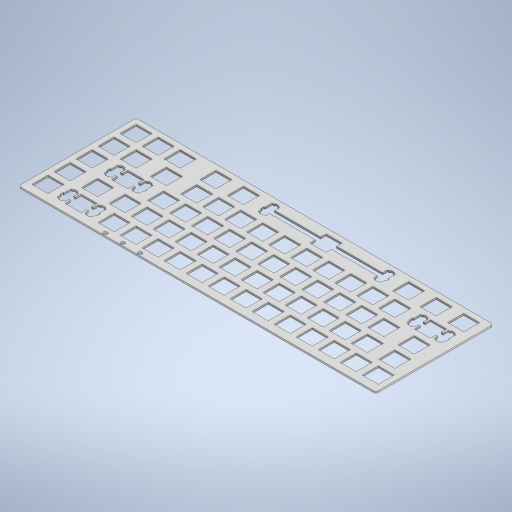
# Autodesk Inventor part: case_plate_p1
Saved by Autodesk Inventor 2024 (Build 280153000, 153)
## iProperties
Created: 2023-08-02
Part Number: case_plate_p1
Material: Generic
Document SubType Name: Modeling
Designer: Mika
Density: 1 g/cm^3
Appearance: Default
Author: Mika
Autodesk Inventor part; units mm, degrees
ref_plane "YZ Plane" through (0, 0, 0) normal (1, 0, 0) x (0, 1, 0)
ref_plane "XZ Plane" through (0, 0, 0) normal (0, 1, 0) x (-1, 0, 0)
ref_plane "XY Plane" through (0, 0, 0) normal (0, 0, 1) x (1, 0, 0)
sketch "Sketch1" plane through (0, 0, 0) normal (0, 1, 0) x (-1, 0, 0)
  line L0 (309.0479, 99.8402) -> (309.0479, 2.3404)
  line L1 (307.045, 0.3402) -> (2.0931, 0.3389)
  line L2 (0.096, 2.3404) -> (0.096, 99.8389)
  line L3 (2.096, 101.8389) -> (307.045, 101.8402)
  line L4 (126.213, 18.8654) -> (126.213, 14.1663)
  line L5 (126.213, 14.1663) -> (86.4387, 14.1663)
  line L6 (86.4387, 14.1663) -> (86.4387, 17.395)
  line L7 (86.4387, 17.395) -> (84.7136, 17.395)
  line L8 (84.7136, 17.395) -> (84.7136, 18.3155)
  line L9 (84.7136, 18.3155) -> (81.5633, 18.3155)
  line L10 (81.5633, 18.3155) -> (81.5633, 17.395)
  line L11 (81.5633, 17.395) -> (79.8382, 17.395)
  line L12 (79.8382, 17.395) -> (79.8382, 14.1663)
  line L13 (79.8382, 14.1663) -> (79.0141, 14.1663)
  line L14 (79.0141, 14.1663) -> (79.0141, 11.5163)
  line L15 (79.0141, 11.5163) -> (79.8382, 11.5163)
  line L16 (79.8382, 11.5163) -> (79.8382, 5.2462)
  line L17 (79.8382, 5.2462) -> (81.5633, 5.2462)
  line L18 (81.5633, 5.2462) -> (81.5633, 4.265)
  line L19 (81.5633, 4.265) -> (84.7136, 4.265)
  line L20 (84.7136, 4.265) -> (84.7136, 5.2462)
  line L21 (84.7136, 5.2462) -> (86.4387, 5.2462)
  line L22 (86.4387, 5.2462) -> (86.4387, 9.7166)
  line L23 (86.4387, 9.7166) -> (126.213, 9.7166)
  line L24 (126.213, 9.7166) -> (126.213, 5.0161)
  line L25 (126.213, 5.0161) -> (140.064, 5.0161)
  line L26 (140.064, 5.0161) -> (140.064, 9.7166)
  line L27 (140.064, 9.7166) -> (179.838, 9.7166)
  line L28 (179.838, 9.7166) -> (179.838, 5.2462)
  line L29 (179.838, 5.2462) -> (181.563, 5.2462)
  line L30 (181.563, 5.2462) -> (181.563, 4.265)
  line L31 (181.563, 4.265) -> (184.714, 4.265)
  line L32 (184.714, 4.265) -> (184.714, 5.2462)
  line L33 (184.714, 5.2462) -> (186.439, 5.2462)
  line L34 (186.439, 5.2462) -> (186.439, 11.5163)
  line L35 (186.439, 11.5163) -> (187.263, 11.5163)
  line L36 (187.263, 11.5163) -> (187.263, 14.1663)
  line L37 (187.263, 14.1663) -> (186.439, 14.1663)
  line L38 (186.439, 14.1663) -> (186.439, 17.395)
  line L39 (186.439, 17.395) -> (184.714, 17.395)
  line L40 (184.714, 17.395) -> (184.714, 18.3155)
  line L41 (184.714, 18.3155) -> (181.563, 18.3155)
  line L42 (181.563, 18.3155) -> (181.563, 17.395)
  line L43 (181.563, 17.395) -> (179.838, 17.395)
  line L44 (179.838, 17.395) -> (179.838, 14.1663)
  line L45 (179.838, 14.1663) -> (140.064, 14.1663)
  line L46 (140.064, 14.1663) -> (140.064, 18.8654)
  line L47 (140.064, 18.8654) -> (126.213, 18.8654)
  line L48 (7.152, 18.8654) -> (21.0013, 18.8654)
  line L49 (21.0013, 18.8654) -> (21.0013, 5.0161)
  line L50 (21.0013, 5.0161) -> (7.152, 5.0161)
  line L51 (7.152, 5.0161) -> (7.152, 18.8654)
  line L52 (30.9631, 18.8654) -> (44.8137, 18.8654)
  line L53 (44.8137, 18.8654) -> (44.8137, 5.0161)
  line L54 (44.8137, 5.0161) -> (30.9631, 5.0161)
  line L55 (30.9631, 5.0161) -> (30.9631, 18.8654)
  line L56 (54.7769, 18.8654) -> (68.6262, 18.8654)
  line L57 (68.6262, 18.8654) -> (68.6262, 5.0161)
  line L58 (68.6262, 5.0161) -> (54.7769, 5.0161)
  line L59 (54.7769, 5.0161) -> (54.7769, 18.8654)
  line L60 (197.652, 18.8654) -> (211.501, 18.8654)
  line L61 (211.501, 18.8654) -> (211.501, 5.0161)
  line L62 (211.501, 5.0161) -> (197.652, 5.0161)
  line L63 (197.652, 5.0161) -> (197.652, 18.8654)
  line L64 (221.463, 18.8654) -> (235.314, 18.8654)
  line L65 (235.314, 18.8654) -> (235.314, 5.0161)
  line L66 (235.314, 5.0161) -> (221.463, 5.0161)
  line L67 (221.463, 5.0161) -> (221.463, 18.8654)
  line L68 (252.421, 18.8654) -> (266.27, 18.8654)
  line L69 (266.27, 18.8654) -> (266.27, 5.0161)
  line L70 (266.27, 5.0161) -> (252.421, 5.0161)
  line L71 (252.421, 5.0161) -> (252.421, 18.8654)
  line L72 (271.471, 18.8654) -> (285.32, 18.8654)
  line L73 (285.32, 18.8654) -> (285.32, 5.0161)
  line L74 (285.32, 5.0161) -> (271.471, 5.0161)
  line L75 (271.471, 5.0161) -> (271.471, 18.8654)
  line L76 (290.521, 18.8654) -> (304.37, 18.8654)
  line L77 (304.37, 18.8654) -> (304.37, 5.0161)
  line L78 (304.37, 5.0161) -> (290.521, 5.0161)
  line L79 (290.521, 5.0161) -> (290.521, 18.8654)
  line L80 (16.677, 37.9155) -> (16.677, 33.2163)
  line L81 (16.677, 33.2163) -> (15.0013, 33.2163)
  line L82 (15.0013, 33.2163) -> (15.0013, 36.4451)
  line L83 (15.0013, 36.4451) -> (13.276, 36.4451)
  line L84 (13.276, 36.4451) -> (13.276, 37.3655)
  line L85 (13.276, 37.3655) -> (10.1258, 37.3655)
  line L86 (10.1258, 37.3655) -> (10.1258, 36.4451)
  line L87 (10.1258, 36.4451) -> (8.4019, 36.4451)
  line L88 (8.4019, 36.4451) -> (8.4019, 33.2163)
  line L89 (8.4019, 33.2163) -> (7.5765, 33.2163)
  line L90 (7.5765, 33.2163) -> (7.5765, 30.5663)
  line L91 (7.5765, 30.5663) -> (8.4019, 30.5663)
  line L92 (8.4019, 30.5663) -> (8.4019, 24.2962)
  line L93 (8.4019, 24.2962) -> (10.1258, 24.2962)
  line L94 (10.1258, 24.2962) -> (10.1258, 23.315)
  line L95 (10.1258, 23.315) -> (13.276, 23.315)
  line L96 (13.276, 23.315) -> (13.276, 24.2962)
  line L97 (13.276, 24.2962) -> (15.0013, 24.2962)
  line L98 (15.0013, 24.2962) -> (15.0013, 28.7652)
  line L99 (15.0013, 28.7652) -> (16.677, 28.7652)
  line L100 (16.677, 28.7652) -> (16.677, 24.0661)
  line L101 (16.677, 24.0661) -> (30.5263, 24.0661)
  line L102 (30.5263, 24.0661) -> (30.5263, 28.7652)
  line L103 (30.5263, 28.7652) -> (32.202, 28.7652)
  line L104 (32.202, 28.7652) -> (32.202, 24.2962)
  line L105 (32.202, 24.2962) -> (33.9259, 24.2962)
  line L106 (33.9259, 24.2962) -> (33.9259, 23.315)
  line L107 (33.9259, 23.315) -> (37.0762, 23.315)
  line L108 (37.0762, 23.315) -> (37.0762, 24.2962)
  line L109 (37.0762, 24.2962) -> (38.8013, 24.2962)
  line L110 (38.8013, 24.2962) -> (38.8013, 30.5663)
  line L111 (38.8013, 30.5663) -> (39.6268, 30.5663)
  line L112 (39.6268, 30.5663) -> (39.6268, 33.2163)
  line L113 (39.6268, 33.2163) -> (38.8013, 33.2163)
  line L114 (38.8013, 33.2163) -> (38.8013, 36.4451)
  line L115 (38.8013, 36.4451) -> (37.0762, 36.4451)
  line L116 (37.0762, 36.4451) -> (37.0762, 37.3655)
  line L117 (37.0762, 37.3655) -> (33.9259, 37.3655)
  line L118 (33.9259, 37.3655) -> (33.9259, 36.4451)
  line L119 (33.9259, 36.4451) -> (32.202, 36.4451)
  line L120 (32.202, 36.4451) -> (32.202, 33.2163)
  line L121 (32.202, 33.2163) -> (30.5263, 33.2163)
  line L122 (30.5263, 33.2163) -> (30.5263, 37.9155)
  line L123 (30.5263, 37.9155) -> (16.677, 37.9155)
  line L124 (47.6321, 37.9155) -> (61.4825, 37.9155)
  line L125 (61.4825, 37.9155) -> (61.4825, 24.0661)
  line L126 (61.4825, 24.0661) -> (47.6321, 24.0661)
  line L127 (47.6321, 24.0661) -> (47.6321, 37.9155)
  line L128 (66.6821, 37.9155) -> (80.5325, 37.9155)
  line L129 (80.5325, 37.9155) -> (80.5325, 24.0661)
  line L130 (80.5325, 24.0661) -> (66.6821, 24.0661)
  line L131 (66.6821, 24.0661) -> (66.6821, 37.9155)
  line L132 (85.7321, 37.9155) -> (99.5825, 37.9155)
  line L133 (99.5825, 37.9155) -> (99.5825, 24.0661)
  line L134 (99.5825, 24.0661) -> (85.7321, 24.0661)
  line L135 (85.7321, 24.0661) -> (85.7321, 37.9155)
  line L136 (104.782, 37.9155) -> (118.632, 37.9155)
  line L137 (118.632, 37.9155) -> (118.632, 24.0661)
  line L138 (118.632, 24.0661) -> (104.782, 24.0661)
  line L139 (104.782, 24.0661) -> (104.782, 37.9155)
  line L140 (123.832, 37.9155) -> (137.682, 37.9155)
  line L141 (137.682, 37.9155) -> (137.682, 24.0661)
  line L142 (137.682, 24.0661) -> (123.832, 24.0661)
  line L143 (123.832, 24.0661) -> (123.832, 37.9155)
  line L144 (142.882, 37.9155) -> (156.732, 37.9155)
  line L145 (156.732, 37.9155) -> (156.732, 24.0661)
  line L146 (156.732, 24.0661) -> (142.882, 24.0661)
  line L147 (142.882, 24.0661) -> (142.882, 37.9155)
  line L148 (161.932, 37.9155) -> (175.782, 37.9155)
  line L149 (175.782, 37.9155) -> (175.782, 24.0661)
  line L150 (175.782, 24.0661) -> (161.932, 24.0661)
  line L151 (161.932, 24.0661) -> (161.932, 37.9155)
  line L152 (180.982, 37.9155) -> (194.832, 37.9155)
  line L153 (194.832, 37.9155) -> (194.832, 24.0661)
  line L154 (194.832, 24.0661) -> (180.982, 24.0661)
  line L155 (180.982, 24.0661) -> (180.982, 37.9155)
  line L156 (200.032, 37.9155) -> (213.882, 37.9155)
  line L157 (213.882, 37.9155) -> (213.882, 24.0661)
  line L158 (213.882, 24.0661) -> (200.032, 24.0661)
  line L159 (200.032, 24.0661) -> (200.032, 37.9155)
  line L160 (219.082, 37.9155) -> (232.932, 37.9155)
  line L161 (232.932, 37.9155) -> (232.932, 24.0661)
  line L162 (232.932, 24.0661) -> (219.082, 24.0661)
  line L163 (219.082, 24.0661) -> (219.082, 37.9155)
  line L164 (245.277, 37.9155) -> (259.126, 37.9155)
  line L165 (259.126, 37.9155) -> (259.126, 24.0661)
  line L166 (259.126, 24.0661) -> (245.277, 24.0661)
  line L167 (245.277, 24.0661) -> (245.277, 37.9155)
  line L168 (271.471, 37.9155) -> (285.32, 37.9155)
  line L169 (285.32, 37.9155) -> (285.32, 24.0661)
  line L170 (285.32, 24.0661) -> (271.471, 24.0661)
  line L171 (271.471, 24.0661) -> (271.471, 37.9155)
  line L172 (290.521, 37.9155) -> (304.37, 37.9155)
  line L173 (304.37, 37.9155) -> (304.37, 24.0661)
  line L174 (304.37, 24.0661) -> (290.521, 24.0661)
  line L175 (290.521, 24.0661) -> (290.521, 37.9155)
  line L176 (259.563, 56.9655) -> (259.563, 52.2661)
  line L177 (259.563, 52.2661) -> (257.889, 52.2661)
  line L178 (257.889, 52.2661) -> (257.889, 55.4951)
  line L179 (257.889, 55.4951) -> (256.162, 55.4951)
  line L180 (256.162, 55.4951) -> (256.162, 56.4155)
  line L181 (256.162, 56.4155) -> (253.013, 56.4155)
  line L182 (253.013, 56.4155) -> (253.013, 55.4951)
  line L183 (253.013, 55.4951) -> (251.288, 55.4951)
  line L184 (251.288, 55.4951) -> (251.288, 52.2661)
  line L185 (251.288, 52.2661) -> (250.464, 52.2661)
  line L186 (250.464, 52.2661) -> (250.464, 49.6164)
  line L187 (250.464, 49.6164) -> (251.288, 49.6164)
  line L188 (251.288, 49.6164) -> (251.288, 43.3462)
  line L189 (251.288, 43.3462) -> (253.013, 43.3462)
  line L190 (253.013, 43.3462) -> (253.013, 42.3651)
  line L191 (253.013, 42.3651) -> (256.162, 42.3651)
  line L192 (256.162, 42.3651) -> (256.162, 43.3462)
  line L193 (256.162, 43.3462) -> (257.889, 43.3462)
  line L194 (257.889, 43.3462) -> (257.889, 47.8151)
  line L195 (257.889, 47.8151) -> (259.563, 47.8151)
  line L196 (259.563, 47.8151) -> (259.563, 43.1161)
  line L197 (259.563, 43.1161) -> (273.414, 43.1161)
  line L198 (273.414, 43.1161) -> (273.414, 47.8151)
  line L199 (273.414, 47.8151) -> (275.088, 47.8151)
  line L200 (275.088, 47.8151) -> (275.088, 43.3462)
  line L201 (275.088, 43.3462) -> (276.813, 43.3462)
  line L202 (276.813, 43.3462) -> (276.813, 42.3651)
  line L203 (276.813, 42.3651) -> (279.964, 42.3651)
  line L204 (279.964, 42.3651) -> (279.964, 43.3462)
  line L205 (279.964, 43.3462) -> (281.689, 43.3462)
  line L206 (281.689, 43.3462) -> (281.689, 49.6164)
  line L207 (281.689, 49.6164) -> (282.513, 49.6164)
  line L208 (282.513, 49.6164) -> (282.513, 52.2661)
  line L209 (282.513, 52.2661) -> (281.689, 52.2661)
  line L210 (281.689, 52.2661) -> (281.689, 55.4951)
  line L211 (281.689, 55.4951) -> (279.964, 55.4951)
  line L212 (279.964, 55.4951) -> (279.964, 56.4155)
  line L213 (279.964, 56.4155) -> (276.813, 56.4155)
  line L214 (276.813, 56.4155) -> (276.813, 55.4951)
  line L215 (276.813, 55.4951) -> (275.088, 55.4951)
  line L216 (275.088, 55.4951) -> (275.088, 52.2661)
  line L217 (275.088, 52.2661) -> (273.414, 52.2661)
  line L218 (273.414, 52.2661) -> (273.414, 56.9655)
  line L219 (273.414, 56.9655) -> (259.563, 56.9655)
  line L220 (11.9131, 56.9655) -> (25.7638, 56.9655)
  line L221 (25.7638, 56.9655) -> (25.7638, 43.1161)
  line L222 (25.7638, 43.1161) -> (11.9131, 43.1161)
  line L223 (11.9131, 43.1161) -> (11.9131, 56.9655)
  line L224 (38.1071, 56.9655) -> (51.9575, 56.9655)
  line L225 (51.9575, 56.9655) -> (51.9575, 43.1161)
  line L226 (51.9575, 43.1161) -> (38.1071, 43.1161)
  line L227 (38.1071, 43.1161) -> (38.1071, 56.9655)
  line L228 (57.1571, 56.9655) -> (71.0075, 56.9655)
  line L229 (71.0075, 56.9655) -> (71.0075, 43.1161)
  line L230 (71.0075, 43.1161) -> (57.1571, 43.1161)
  line L231 (57.1571, 43.1161) -> (57.1571, 56.9655)
  line L232 (76.2071, 56.9655) -> (90.0575, 56.9655)
  line L233 (90.0575, 56.9655) -> (90.0575, 43.1161)
  line L234 (90.0575, 43.1161) -> (76.2071, 43.1161)
  line L235 (76.2071, 43.1161) -> (76.2071, 56.9655)
  line L236 (95.2571, 56.9655) -> (109.107, 56.9655)
  line L237 (109.107, 56.9655) -> (109.107, 43.1161)
  line L238 (109.107, 43.1161) -> (95.2571, 43.1161)
  line L239 (95.2571, 43.1161) -> (95.2571, 56.9655)
  line L240 (114.307, 56.9655) -> (128.157, 56.9655)
  line L241 (128.157, 56.9655) -> (128.157, 43.1161)
  line L242 (128.157, 43.1161) -> (114.307, 43.1161)
  line L243 (114.307, 43.1161) -> (114.307, 56.9655)
  line L244 (133.357, 56.9655) -> (147.207, 56.9655)
  line L245 (147.207, 56.9655) -> (147.207, 43.1161)
  line L246 (147.207, 43.1161) -> (133.357, 43.1161)
  line L247 (133.357, 43.1161) -> (133.357, 56.9655)
  line L248 (152.407, 56.9655) -> (166.257, 56.9655)
  line L249 (166.257, 56.9655) -> (166.257, 43.1161)
  line L250 (166.257, 43.1161) -> (152.407, 43.1161)
  line L251 (152.407, 43.1161) -> (152.407, 56.9655)
  line L252 (171.457, 56.9655) -> (185.307, 56.9655)
  line L253 (185.307, 56.9655) -> (185.307, 43.1161)
  line L254 (185.307, 43.1161) -> (171.457, 43.1161)
  line L255 (171.457, 43.1161) -> (171.457, 56.9655)
  line L256 (190.507, 56.9655) -> (204.357, 56.9655)
  line L257 (204.357, 56.9655) -> (204.357, 43.1161)
  line L258 (204.357, 43.1161) -> (190.507, 43.1161)
  line L259 (190.507, 43.1161) -> (190.507, 56.9655)
  line L260 (209.557, 56.9655) -> (223.407, 56.9655)
  line L261 (223.407, 56.9655) -> (223.407, 43.1161)
  line L262 (223.407, 43.1161) -> (209.557, 43.1161)
  line L263 (209.557, 43.1161) -> (209.557, 56.9655)
  line L264 (228.607, 56.9655) -> (242.457, 56.9655)
  line L265 (242.457, 56.9655) -> (242.457, 43.1161)
  line L266 (242.457, 43.1161) -> (228.607, 43.1161)
  line L267 (228.607, 43.1161) -> (228.607, 56.9655)
  line L268 (290.521, 56.9655) -> (304.37, 56.9655)
  line L269 (304.37, 56.9655) -> (304.37, 43.1161)
  line L270 (304.37, 43.1161) -> (290.521, 43.1161)
  line L271 (290.521, 43.1161) -> (290.521, 56.9655)
  line L272 (9.5319, 76.0155) -> (23.3826, 76.0155)
  line L273 (23.3826, 76.0155) -> (23.3826, 62.1661)
  line L274 (23.3826, 62.1661) -> (9.5319, 62.1661)
  line L275 (9.5319, 62.1661) -> (9.5319, 76.0155)
  line L276 (33.3458, 76.0155) -> (47.195, 76.0155)
  line L277 (47.195, 76.0155) -> (47.195, 62.1661)
  line L278 (47.195, 62.1661) -> (33.3458, 62.1661)
  line L279 (33.3458, 62.1661) -> (33.3458, 76.0155)
  line L280 (52.3956, 76.0155) -> (66.245, 76.0155)
  line L281 (66.245, 76.0155) -> (66.245, 62.1661)
  line L282 (66.245, 62.1661) -> (52.3956, 62.1661)
  line L283 (52.3956, 62.1661) -> (52.3956, 76.0155)
  line L284 (71.4456, 76.0155) -> (85.295, 76.0155)
  line L285 (85.295, 76.0155) -> (85.295, 62.1661)
  line L286 (85.295, 62.1661) -> (71.4456, 62.1661)
  line L287 (71.4456, 62.1661) -> (71.4456, 76.0155)
  line L288 (90.4946, 76.0155) -> (104.345, 76.0155)
  line L289 (104.345, 76.0155) -> (104.345, 62.1661)
  line L290 (104.345, 62.1661) -> (90.4946, 62.1661)
  line L291 (90.4946, 62.1661) -> (90.4946, 76.0155)
  line L292 (109.545, 76.0155) -> (123.395, 76.0155)
  line L293 (123.395, 76.0155) -> (123.395, 62.1661)
  line L294 (123.395, 62.1661) -> (109.545, 62.1661)
  line L295 (109.545, 62.1661) -> (109.545, 76.0155)
  line L296 (128.595, 76.0155) -> (142.445, 76.0155)
  line L297 (142.445, 76.0155) -> (142.445, 62.1661)
  line L298 (142.445, 62.1661) -> (128.595, 62.1661)
  line L299 (128.595, 62.1661) -> (128.595, 76.0155)
  line L300 (147.645, 76.0155) -> (161.495, 76.0155)
  line L301 (161.495, 76.0155) -> (161.495, 62.1661)
  line L302 (161.495, 62.1661) -> (147.645, 62.1661)
  line L303 (147.645, 62.1661) -> (147.645, 76.0155)
  line L304 (166.696, 76.0155) -> (180.545, 76.0155)
  line L305 (180.545, 76.0155) -> (180.545, 62.1661)
  line L306 (180.545, 62.1661) -> (166.696, 62.1661)
  line L307 (166.696, 62.1661) -> (166.696, 76.0155)
  line L308 (185.746, 76.0155) -> (199.595, 76.0155)
  line L309 (199.595, 76.0155) -> (199.595, 62.1661)
  line L310 (199.595, 62.1661) -> (185.746, 62.1661)
  line L311 (185.746, 62.1661) -> (185.746, 76.0155)
  line L312 (204.796, 76.0155) -> (218.645, 76.0155)
  line L313 (218.645, 76.0155) -> (218.645, 62.1661)
  line L314 (218.645, 62.1661) -> (204.796, 62.1661)
  line L315 (204.796, 62.1661) -> (204.796, 76.0155)
  line L316 (223.846, 76.0155) -> (237.695, 76.0155)
  line L317 (237.695, 76.0155) -> (237.695, 62.1661)
  line L318 (237.695, 62.1661) -> (223.846, 62.1661)
  line L319 (223.846, 62.1661) -> (223.846, 76.0155)
  line L320 (242.896, 76.0155) -> (256.745, 76.0155)
  line L321 (256.745, 76.0155) -> (256.745, 62.1661)
  line L322 (256.745, 62.1661) -> (242.896, 62.1661)
  line L323 (242.896, 62.1661) -> (242.896, 76.0155)
  line L324 (266.707, 76.0155) -> (280.557, 76.0155)
  line L325 (280.557, 76.0155) -> (280.557, 62.1661)
  line L326 (280.557, 62.1661) -> (266.707, 62.1661)
  line L327 (266.707, 62.1661) -> (266.707, 76.0155)
  line L328 (290.521, 76.0155) -> (304.37, 76.0155)
  line L329 (304.37, 76.0155) -> (304.37, 62.1661)
  line L330 (304.37, 62.1661) -> (290.521, 62.1661)
  line L331 (290.521, 62.1661) -> (290.521, 76.0155)
  line L332 (261.946, 95.0655) -> (261.946, 90.3661)
  line L333 (261.946, 90.3661) -> (260.27, 90.3661)
  line L334 (260.27, 90.3661) -> (260.27, 93.5951)
  line L335 (260.27, 93.5951) -> (258.546, 93.5951)
  line L336 (258.546, 93.5951) -> (258.546, 94.5155)
  line L337 (258.546, 94.5155) -> (255.396, 94.5155)
  line L338 (255.396, 94.5155) -> (255.396, 93.5951)
  line L339 (255.396, 93.5951) -> (253.67, 93.5951)
  line L340 (253.67, 93.5951) -> (253.67, 90.3661)
  line L341 (253.67, 90.3661) -> (252.845, 90.3661)
  line L342 (252.845, 90.3661) -> (252.845, 87.7164)
  line L343 (252.845, 87.7164) -> (253.67, 87.7164)
  line L344 (253.67, 87.7164) -> (253.67, 81.4462)
  line L345 (253.67, 81.4462) -> (255.396, 81.4462)
  line L346 (255.396, 81.4462) -> (255.396, 80.4651)
  line L347 (255.396, 80.4651) -> (258.546, 80.4651)
  line L348 (258.546, 80.4651) -> (258.546, 81.4462)
  line L349 (258.546, 81.4462) -> (260.27, 81.4462)
  line L350 (260.27, 81.4462) -> (260.27, 85.9151)
  line L351 (260.27, 85.9151) -> (261.946, 85.9151)
  line L352 (261.946, 85.9151) -> (261.946, 81.2161)
  line L353 (261.946, 81.2161) -> (275.795, 81.2161)
  line L354 (275.795, 81.2161) -> (275.795, 85.9151)
  line L355 (275.795, 85.9151) -> (277.471, 85.9151)
  line L356 (277.471, 85.9151) -> (277.471, 81.4462)
  line L357 (277.471, 81.4462) -> (279.196, 81.4462)
  line L358 (279.196, 81.4462) -> (279.196, 80.4651)
  line L359 (279.196, 80.4651) -> (282.345, 80.4651)
  line L360 (282.345, 80.4651) -> (282.345, 81.4462)
  line L361 (282.345, 81.4462) -> (284.07, 81.4462)
  line L362 (284.07, 81.4462) -> (284.07, 87.7164)
  line L363 (284.07, 87.7164) -> (284.896, 87.7164)
  line L364 (284.896, 87.7164) -> (284.896, 90.3661)
  line L365 (284.896, 90.3661) -> (284.07, 90.3661)
  line L366 (284.07, 90.3661) -> (284.07, 93.5951)
  line L367 (284.07, 93.5951) -> (282.345, 93.5951)
  line L368 (282.345, 93.5951) -> (282.345, 94.5155)
  line L369 (282.345, 94.5155) -> (279.196, 94.5155)
  line L370 (279.196, 94.5155) -> (279.196, 93.5951)
  line L371 (279.196, 93.5951) -> (277.471, 93.5951)
  line L372 (277.471, 93.5951) -> (277.471, 90.3661)
  line L373 (277.471, 90.3661) -> (275.795, 90.3661)
  line L374 (275.795, 90.3661) -> (275.795, 95.0655)
  line L375 (275.795, 95.0655) -> (261.946, 95.0655)
  line L376 (4.7708, 95.0655) -> (18.6201, 95.0655)
  line L377 (18.6201, 95.0655) -> (18.6201, 81.2161)
  line L378 (18.6201, 81.2161) -> (4.7708, 81.2161)
  line L379 (4.7708, 81.2161) -> (4.7708, 95.0655)
  line L380 (23.8208, 95.0655) -> (37.67, 95.0655)
  line L381 (37.67, 95.0655) -> (37.67, 81.2161)
  line L382 (37.67, 81.2161) -> (23.8208, 81.2161)
  line L383 (23.8208, 81.2161) -> (23.8208, 95.0655)
  line L384 (42.8706, 95.0655) -> (56.72, 95.0655)
  line L385 (56.72, 95.0655) -> (56.72, 81.2161)
  line L386 (56.72, 81.2161) -> (42.8706, 81.2161)
  line L387 (42.8706, 81.2161) -> (42.8706, 95.0655)
  line L388 (61.9206, 95.0655) -> (75.77, 95.0655)
  line L389 (75.77, 95.0655) -> (75.77, 81.2161)
  line L390 (75.77, 81.2161) -> (61.9206, 81.2161)
  line L391 (61.9206, 81.2161) -> (61.9206, 95.0655)
  line L392 (80.9706, 95.0655) -> (94.82, 95.0655)
  line L393 (94.82, 95.0655) -> (94.82, 81.2161)
  line L394 (94.82, 81.2161) -> (80.9706, 81.2161)
  line L395 (80.9706, 81.2161) -> (80.9706, 95.0655)
  line L396 (100.021, 95.0655) -> (113.87, 95.0655)
  line L397 (113.87, 95.0655) -> (113.87, 81.2161)
  line L398 (113.87, 81.2161) -> (100.021, 81.2161)
  line L399 (100.021, 81.2161) -> (100.021, 95.0655)
  line L400 (119.071, 95.0655) -> (132.92, 95.0655)
  line L401 (132.92, 95.0655) -> (132.92, 81.2161)
  line L402 (132.92, 81.2161) -> (119.071, 81.2161)
  line L403 (119.071, 81.2161) -> (119.071, 95.0655)
  line L404 (138.121, 95.0655) -> (151.97, 95.0655)
  line L405 (151.97, 95.0655) -> (151.97, 81.2161)
  line L406 (151.97, 81.2161) -> (138.121, 81.2161)
  line L407 (138.121, 81.2161) -> (138.121, 95.0655)
  line L408 (157.171, 95.0655) -> (171.02, 95.0655)
  line L409 (171.02, 95.0655) -> (171.02, 81.2161)
  line L410 (171.02, 81.2161) -> (157.171, 81.2161)
  line L411 (157.171, 81.2161) -> (157.171, 95.0655)
  line L412 (176.221, 95.0655) -> (190.07, 95.0655)
  line L413 (190.07, 95.0655) -> (190.07, 81.2161)
  line L414 (190.07, 81.2161) -> (176.221, 81.2161)
  line L415 (176.221, 81.2161) -> (176.221, 95.0655)
  line L416 (195.271, 95.0655) -> (209.12, 95.0655)
  line L417 (209.12, 95.0655) -> (209.12, 81.2161)
  line L418 (209.12, 81.2161) -> (195.271, 81.2161)
  line L419 (195.271, 81.2161) -> (195.271, 95.0655)
  line L420 (214.321, 95.0655) -> (228.17, 95.0655)
  line L421 (228.17, 95.0655) -> (228.17, 81.2161)
  line L422 (228.17, 81.2161) -> (214.321, 81.2161)
  line L423 (214.321, 81.2161) -> (214.321, 95.0655)
  line L424 (233.371, 95.0655) -> (247.22, 95.0655)
  line L425 (247.22, 95.0655) -> (247.22, 81.2161)
  line L426 (247.22, 81.2161) -> (233.371, 81.2161)
  line L427 (233.371, 81.2161) -> (233.371, 95.0655)
  line L428 (290.521, 95.0655) -> (304.37, 95.0655)
  line L429 (304.37, 95.0655) -> (304.37, 81.2161)
  line L430 (304.37, 81.2161) -> (290.521, 81.2161)
  line L431 (290.521, 81.2161) -> (290.521, 95.0655)
  arc A0 (307.045, 0.3402) -> (309.0479, 2.3404) centre (307.0479, 2.3402) ccw
  arc A1 (0.096, 2.3404) -> (2.0931, 0.3389) centre (2.096, 2.3389) ccw
  arc A2 (309.0479, 99.8402) -> (307.045, 101.8402) centre (307.0479, 99.8402) ccw
  arc A3 (2.096, 101.8389) -> (0.096, 99.8389) centre (2.096, 99.8389) ccw
  line L432 (221.0479, 101.8399) -> (221.0479, 99.8399)
  line L433 (221.0479, 99.8399) -> (236.0479, 99.8399)
  line L434 (221.0479, 99.8399) -> (206.0479, 99.8399)
  line L435 (221.0479, 99.8399) -> (236.0479, 99.8399) construction
  circle A4 centre (221.0479, 99.8399) radius 1.75
  circle A5 centre (206.0479, 99.8399) radius 1.75
  circle A6 centre (236.0479, 99.8399) radius 1.75
  line L436 (193.4145, 0.3397) -> (193.4145, 20.9073)
  line L437 (193.4145, 20.9073) -> (178.382, 20.9073)
  line L438 (178.382, 20.9073) -> (178.382, 40.376)
  line L439 (178.382, 40.376) -> (187.907, 40.376)
  line L440 (187.907, 40.376) -> (187.907, 59.7445)
  line L441 (187.907, 59.7445) -> (183.1445, 59.7445)
  line L442 (183.1445, 59.7445) -> (183.1445, 78.7061)
  line L443 (183.1445, 78.7061) -> (192.6705, 78.7061)
  line L444 (192.6705, 78.7061) -> (192.6704, 101.8397)
  point P0 (4.7708, 81.2161)
  point P1 (7.152, 5.0161)
  dimension "d0" = 308.9519
  dimension "d1" = 101.5
  dimension "d12" = 88
  dimension "d13" = 2
  dimension "d14" = 15
  dimension "d15" = 15
  dimension "d16" = 180
  dimension "d20" = 3.5
  dimension "d21" = 3.5
  dimension "d22" = 3.5
  constraints: 896 end point, 8 point on circle, 7 centre point, 7 perpendicular, 4 coincident, 4 horizontal, 3 point on line, 2 vertical, 1 collinear, 1 parallel
  measures "d0" distance between parallel lines of L0 L2
  measures "d1" distance between parallel lines of L3 L1
  measures "d12" distance from line of L0.start L432
  measures "d13" distance of L432.start L432.end
  measures "d14" distance of L433.start L433.end
  measures "d15" distance of L433.start L434.end
  measures "d16" angle of L434 L435
  measures "d20" diameter of A4
  measures "d21" diameter of A5
  measures "d22" diameter of A6
extrude "Extrusion1" add sketch "Sketch1" along normal blind 1.48 contours L0 A0 L1 L436 L437 L438 L439 L440 L441 L442 L443 L444 L3 A2 | L1 A1 L2 A3 L3 L444 L443 L442 L441 L440 L439 L438 L437 L436 | A4 L433 L432 | L432 L434 A4 | L433 A4 L434 | A5 | A6
extrude "Extrusion2" cut sketch "Sketch1" along normal blind 1.48 contours A4 L433 L432 | L432 L434 A4 | L433 A4 L434 | A5 | A6
body "Solid1"
